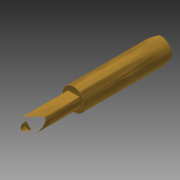
# Autodesk Inventor part: shaft
Saved by Autodesk Inventor 2014 (Build 180170000, 170)
## iProperties
Shininess: 27.0
Length Units: 11272
Angle Units: 11279
Time Units: 11290
Mass Units: 11286
Length Display Precision: 3
Angle Display Precision: 2
Compacted: True
Created: 2001-07-10
Part Number: shaft
Document SubType Name: Modeling
Designer: Autodesk, Inc.
Mass: 11.6627 g
Surface Area: 9.74768 cm^2
Volume: 1.37694 cm^3
Density: 8.47 g/cm^3
Material: Brass, Soft Yellow
Appearance: Brass - Satin
Density: 0.0
Volumn: 0.0
Area: 0.0
PropertySet Name: Model Information
Control State: 0
Master: False
Checked Out: False
Author: Autodesk, Inc.
Autodesk Inventor part; units mm, degrees
ref_plane "YZ Plane" through (0, 0, 0) normal (1, 0, 0) x (0, 1, 0)
ref_plane "XZ Plane" through (0, 0, 0) normal (0, 1, 0) x (-1, 0, 0)
ref_plane "XY Plane" through (0, 0, 0) normal (0, 0, 1) x (1, 0, 0)
sketch "Sketch1" plane through (0, 0, 0) normal (0, 0, 1) x (1, 0, 0)
  circle A0 centre (0, 0) radius 3.5719
  dimension "d10" = 7.1437
  constraints: 1 centre point
  measures "d10" diameter of A0
extrude "Extrusion1" add sketch "Sketch1" along normal blind 45.2438
sketch "Sketch2" plane through (0, 0, 45.2438) normal (0, 0, 1) x (1, 0, 0)
  arc A0 (-1.7749, 1.5875) -> (1.7749, 1.5875) centre (0, 0) ccw
  line L0 (1.7749, 1.5875) -> (-1.7749, 1.5875)
  circle A1 centre (0, 0) radius 3.5719 projected
  dimension "d2" = 4.7625
  constraints: 2 end point, 2 point on circle, 1 centre point, 1 horizontal
  measures "d2" diameter of A0
extrude "Extrusion2" cut sketch "Sketch2" against normal blind 17.4625
sketch "Sketch3" plane through (0, 0, 45.2438) normal (0, 0, 1) x (1, 0, 0)
  circle A0 centre (0, 0) radius 1.143
  dimension "d5" = 2.286
  constraints: 1 centre point
  measures "d5" diameter of A0
extrude "Extrusion3" cut sketch "Sketch3" against normal blind 3.175
chamfer "Chamfer1" distance 0.127 angle 45 5 edges at (0, -2.3813, 45.2438) (0, 1.5875, 45.2438) (-1.143, 0, 45.2438) (-3.5719, 0, 27.7813) (-3.5719, 0, 0)
body "Solid1"
